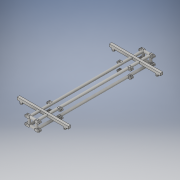
# Autodesk Inventor part: prototype body
Saved by Autodesk Inventor 2016 (Build 200138000, 138)
## iProperties
Created: 2017-06-26
Part Number: prototype body
Material: Generic
Document SubType Name: Modeling
Designer: andon
Density: 1 g/cm^3
Appearance: Default
Author: andon
Autodesk Inventor part; units mm, degrees
sketch "Sketch1" plane through (0, 0, 0) normal (0, 0, 1) x (1, 0, 0)
  line L0 (-76.2, -76.2) -> (76.2, -76.2)
  line L1 (76.2, -76.2) -> (76.2, 76.2)
  line L2 (76.2, 76.2) -> (-76.2, 76.2)
  line L3 (-76.2, 76.2) -> (-76.2, -76.2)
  line L4 (-76.2, -76.2) -> (76.2, 76.2) construction
  line L5 (76.2, -76.2) -> (-76.2, 76.2) construction
  circle A0 centre (-76.2, 76.2) radius 25.4
  circle A1 centre (76.2, 76.2) radius 25.4
  circle A2 centre (-76.2, -76.2) radius 25.4
  circle A3 centre (76.2, -76.2) radius 25.4
  point P0 (0, 0)
  dimension "d0" = 152.4
  dimension "d1" = 152.4
  dimension "d6" = 50.8
  constraints: 12 end point, 4 centre point, 4 coincident, 3 equal radius, 2 midpoint, 2 parallel, 1 horizontal, 1 perpendicular
  measures "d0" distance of L2.end L1.end
  measures "d1" distance of L1.end L0.end
  measures "d6" diameter of A1
sketch "Sketch1 outline for Extrusion1" plane through (0, 0, 0) normal (0, 0, 1) x (1, 0, 0)
  circle A0 centre (-76.2, 76.2) radius 25.4
  circle A1 centre (76.2, 76.2) radius 25.4
  circle A2 centre (-76.2, -76.2) radius 25.4
  circle A3 centre (76.2, -76.2) radius 25.4
extrude "Extrusion1" add sketch "Sketch1 outline for Extrusion1" along normal mid plane 2438.4
sketch "Sketch2" plane through (-76.2, 76.2, 1219.2) normal (0, 0, 1) x (1, 0, 0)
  circle A0 centre (0, 0) radius 25.4 projected
  circle A1 centre (0, -152.4) radius 25.4 projected
  circle A2 centre (152.4, 0) radius 25.4 projected
  circle A3 centre (152.4, -152.4) radius 25.4 projected
  line L0 (0, 0) -> (152.4, 0)
  line L1 (152.4, 0) -> (152.4, -152.4)
  line L2 (152.4, -152.4) -> (0, -152.4)
  line L3 (0, -152.4) -> (0, 0)
  point P0 (76.2, -76.2)
  constraints: 8 end point, 2 parallel, 1 horizontal, 1 perpendicular
ref_plane "Work Plane1" through (76.2, 76.2, 1219.2) normal (-1, 0, 0) x (0, -1, 0)
sketch "Sketch3" plane through (76.2, 76.2, 1219.2) normal (-1, 0, 0) x (0, -1, 0)
  circle A0 centre (0, -25.4) radius 25.4
  circle A1 centre (152.4, -25.4) radius 25.4
  line L0 (25.4, -1219.2) -> (-25.4, -1219.2) projected
  line L1 (25.4, -1219.2) -> (-25.4, -1219.2) projected
  line L2 (177.8, -1219.2) -> (127, -1219.2) projected
  circle A2 centre (152.4, -2413) radius 25.4
  line L3 (127, -2438.4) -> (127, 0) projected
  circle A3 centre (0, -2413) radius 25.4
  line L4 (-25.4, -2438.4) -> (-25.4, 0) projected
  point P0 (76.2, -1219.2)
  dimension "d10" = 50.8
  constraints: 4 centre point, 2 tangent, 1 equal radius
  measures "d10" diameter of A0
sketch "Sketch3 outline for Extrusion2" plane through (76.2, 76.2, 1219.2) normal (-1, 0, 0) x (0, -1, 0)
  circle A0 centre (0, -25.4) radius 25.4
  circle A1 centre (152.4, -25.4) radius 25.4
  circle A2 centre (152.4, -2413) radius 25.4
  circle A3 centre (0, -2413) radius 25.4
extrude "Extrusion2" add sketch "Sketch3 outline for Extrusion2" along normal blind 152.4
ref_plane "Work Plane2" through (-76.2, 76.2, 1219.2) normal (0, -1, 0) x (1, 0, 0)
sketch "Sketch4" plane through (-76.2, 76.2, 1219.2) normal (0, -1, 0) x (1, 0, 0)
  line L0 (0, -25.4) -> (25.4, -50.8) projected
  circle A0 centre (0, -25.4) radius 25.4
  line L1 (152.4, -25.4) -> (127, 0) projected
  circle A1 centre (152.4, -25.4) radius 25.4
  line L2 (0, -1803.4) -> (0, -1803.4) projected
  line L3 (152.4, -1803.4) -> (127, -1778) projected
  circle A2 centre (0, -2413) radius 25.4
  line L4 (-25.4, -2438.4) -> (25.4, -2438.4) projected
  line L5 (152.4, -2413) -> (127, -2387.6) projected
  circle A3 centre (152.4, -2413) radius 25.4
  point P0 (76.2, -1219.2)
  dimension "d14" = 50.8
  constraints: 4 centre point, 1 equal radius, 1 tangent, 1 other
  measures "d14" diameter of A0
sketch "Sketch4 outline for Extrusion3" plane through (-76.2, 76.2, 1219.2) normal (0, -1, 0) x (1, 0, 0)
  circle A0 centre (0, -25.4) radius 25.4
  circle A1 centre (152.4, -25.4) radius 25.4
  circle A2 centre (0, -2413) radius 25.4
  circle A3 centre (152.4, -2413) radius 25.4
extrude "Extrusion3" add sketch "Sketch4 outline for Extrusion3" along normal blind 152.4
ref_plane "Work Plane3" through (0, 76.2, 1219.2) normal (-1, 0, 0) x (0, -1, 0)
sketch "Sketch7" plane through (0, 76.2, 1219.2) normal (-1, 0, 0) x (0, -1, 0)
  line L0 (-25.4, -228.6) -> (25.4, -228.6)
  line L1 (25.4, -228.6) -> (25.4, -279.4)
  line L2 (25.4, -279.4) -> (-25.4, -279.4)
  line L3 (-25.4, -279.4) -> (-25.4, -228.6)
  line L4 (-25.4, -228.6) -> (25.4, -279.4) construction
  line L5 (25.4, -228.6) -> (-25.4, -279.4) construction
  point P0 (76.2, -1219.2)
  point P1 (0, -254)
  dimension "d23" = 50.8
  dimension "d24" = 50.8
  constraints: 12 end point, 2 midpoint, 2 parallel, 1 horizontal, 1 perpendicular
  measures "d23" distance of L1.end L2.end
  measures "d24" distance of L0.end L1.end
sketch "Sketch7 outline for Extrusion4" plane through (0, 76.2, 1219.2) normal (-1, 0, 0) x (0, -1, 0)
  line L0 (-25.4, -228.6) -> (25.4, -228.6)
  line L1 (25.4, -228.6) -> (25.4, -279.4)
  line L2 (25.4, -279.4) -> (-25.4, -279.4)
  line L3 (-25.4, -279.4) -> (-25.4, -228.6)
extrude "Extrusion4" add sketch "Sketch7 outline for Extrusion4" along normal mid plane 1066.8
sketch "Sketch9" plane through (76.2, 76.2, 1219.2) normal (-1, 0, 0) x (0, -1, 0)
  line L0 (0, -25.4) -> (25.4, -50.8) projected
  line L1 (-25.4, 0) -> (25.4, 0)
  line L2 (25.4, 0) -> (25.4, -50.8)
  line L3 (25.4, -50.8) -> (-25.4, -50.8)
  line L4 (-25.4, -50.8) -> (-25.4, 0)
  line L5 (-25.4, 0) -> (25.4, -50.8) construction
  line L6 (25.4, 0) -> (-25.4, -50.8) construction
  line L7 (127, 0) -> (177.8, 0)
  line L8 (177.8, 0) -> (177.8, -50.8)
  line L9 (177.8, -50.8) -> (127, -50.8)
  line L10 (127, -50.8) -> (127, 0)
  line L11 (152.4, -25.4) -> (127, 0) projected
  line L12 (127, 0) -> (177.8, -50.8) construction
  line L13 (177.8, 0) -> (127, -50.8) construction
  line L14 (-50.8, -25.4) -> (-50.8, -482.6)
  line L15 (-25.4, -457.2) -> (25.4, -457.2)
  line L16 (25.4, -457.2) -> (25.4, -508)
  line L17 (25.4, -508) -> (-25.4, -508)
  line L18 (-25.4, -508) -> (-25.4, -457.2)
  line L19 (-25.4, -457.2) -> (25.4, -508) construction
  line L20 (25.4, -457.2) -> (-25.4, -508) construction
  line L21 (127, -457.2) -> (177.8, -457.2)
  line L22 (177.8, -457.2) -> (177.8, -508)
  line L23 (177.8, -508) -> (127, -508)
  line L24 (127, -508) -> (127, -457.2)
  line L25 (127, -457.2) -> (177.8, -508) construction
  line L26 (177.8, -457.2) -> (127, -508) construction
  point P0 (76.2, -1219.2)
  point P1 (17.960512, -43.360512)
  point P2 (0, -482.6)
  point P3 (152.4, -482.6)
  dimension "d27" = 50.8
  dimension "d28" = 50.8
  dimension "d29" = 50.8
  dimension "d30" = 50.8
  dimension "d31" = 457.2
  dimension "d32" = 50.8
  dimension "d33" = 50.8
  dimension "d34" = 50.8
  dimension "d35" = 50.8
  constraints: 50 end point, 8 midpoint, 8 parallel, 4 horizontal, 4 perpendicular, 1 vertical
  measures "d27" distance of L0.end L3.end
  measures "d28" distance of L1.end L0.end
  measures "d29" distance of L8.end L9.end
  measures "d30" distance of L7.end L8.end
  measures "d31" distance of L14.start L14.end
  measures "d32" distance of L16.end L17.end
  measures "d33" distance of L15.end L16.end
  measures "d34" distance of L22.end L23.end
  measures "d35" distance of L21.end L22.end
sketch "Sketch9 outline for Extrusion5" plane through (76.2, 76.2, 1219.2) normal (-1, 0, 0) x (0, -1, 0)
  line L0 (-25.4, 0) -> (25.4, 0)
  line L1 (25.4, 0) -> (25.4, -50.8)
  line L2 (25.4, -50.8) -> (-25.4, -50.8)
  line L3 (-25.4, -50.8) -> (-25.4, 0)
  line L4 (127, 0) -> (177.8, 0)
  line L5 (177.8, 0) -> (177.8, -50.8)
  line L6 (177.8, -50.8) -> (127, -50.8)
  line L7 (127, -50.8) -> (127, 0)
  line L8 (-25.4, -457.2) -> (25.4, -457.2)
  line L9 (25.4, -457.2) -> (25.4, -508)
  line L10 (25.4, -508) -> (-25.4, -508)
  line L11 (-25.4, -508) -> (-25.4, -457.2)
  line L12 (127, -457.2) -> (177.8, -457.2)
  line L13 (177.8, -457.2) -> (177.8, -508)
  line L14 (177.8, -508) -> (127, -508)
  line L15 (127, -508) -> (127, -457.2)
extrude "Extrusion5" add sketch "Sketch9 outline for Extrusion5" against normal blind 76.2
sketch "Sketch10" plane through (152.4, 76.2, 1219.2) normal (1, 0, 0) x (0, 0, -1)
  line L0 (50.8, 25.4) -> (0, 25.4) projected
  line L1 (0, -25.4) -> (50.8, -25.4) projected
  line L2 (12.7, 25.4) -> (38.1, 25.4)
  line L3 (38.1, 25.4) -> (38.1, -25.4)
  line L4 (38.1, -25.4) -> (12.7, -25.4)
  line L5 (12.7, -25.4) -> (12.7, 25.4)
  line L6 (50.8, -127) -> (0, -127) projected
  line L7 (2438.4, -177.8) -> (0, -177.8) projected
  line L8 (12.7, -127) -> (38.1, -127)
  line L9 (38.1, -127) -> (38.1, -177.8)
  line L10 (38.1, -177.8) -> (12.7, -177.8)
  line L11 (12.7, -177.8) -> (12.7, -127)
  line L12 (2387.6, -127) -> (50.8, -127) projected
  line L13 (469.9, -127) -> (495.3, -127)
  line L14 (495.3, -127) -> (495.3, -177.8)
  line L15 (495.3, -177.8) -> (469.9, -177.8)
  line L16 (469.9, -177.8) -> (469.9, -127)
  line L17 (2387.6, -25.4) -> (279.4, -25.4) projected
  line L18 (469.9, 25.4) -> (495.3, 25.4)
  line L19 (495.3, 25.4) -> (495.3, -25.4)
  line L20 (495.3, -25.4) -> (469.9, -25.4)
  line L21 (469.9, -25.4) -> (469.9, 25.4)
  point P0 (1219.2, -76.2)
  constraints: 32 end point, 12 point on line, 8 parallel, 4 horizontal, 4 perpendicular
sketch "Sketch10 outline for Extrusion6" plane through (152.4, 76.2, 1219.2) normal (1, 0, 0) x (0, 0, -1)
  line L0 (12.7, 25.4) -> (38.1, 25.4)
  line L1 (38.1, 25.4) -> (38.1, -25.4)
  line L2 (38.1, -25.4) -> (12.7, -25.4)
  line L3 (12.7, -25.4) -> (12.7, 25.4)
  line L4 (469.9, 25.4) -> (495.3, 25.4)
  line L5 (495.3, 25.4) -> (495.3, -25.4)
  line L6 (495.3, -25.4) -> (469.9, -25.4)
  line L7 (469.9, -25.4) -> (469.9, 25.4)
  line L8 (469.9, -177.8) -> (495.3, -177.8)
  line L9 (469.9, -127) -> (469.9, -177.8)
  line L10 (495.3, -127) -> (469.9, -127)
  line L11 (495.3, -177.8) -> (495.3, -127)
  line L12 (38.1, -127) -> (12.7, -127)
  line L13 (38.1, -177.8) -> (38.1, -127)
  line L14 (12.7, -177.8) -> (38.1, -177.8)
  line L15 (12.7, -127) -> (12.7, -177.8)
extrude "Extrusion6" cut sketch "Sketch10 outline for Extrusion6" against normal blind 50.8
fillet "Fillet1" radius 25.4 16 edges at (152.4, 101.6, 1212.85) (152.4, 50.8, 1212.85) (152.4, 50.8, 1174.75) (152.4, 101.6, 1174.75) (152.4, -50.8, 1174.75) (152.4, -101.6, 1174.75) (152.4, -101.6, 1212.85) (152.4, -50.8, 1212.85) (152.4, 101.6, 755.65) (152.4, 101.6, 717.55) (152.4, 50.8, 717.55) (152.4, 50.8, 755.65) (152.4, -50.8, 755.65) (152.4, -50.8, 717.55) (152.4, -101.6, 717.55) (152.4, -101.6, 755.65)
sketch "Sketch11" plane through (0, 0, 1219.2) normal (0, 0, 1) x (1, 0, 0)
  arc A0 (127, 50.8) -> (127, 101.6) centre (127, 76.2) ccw projected
  circle A1 centre (127, 76.2) radius 9.525
  circle A2 centre (127, -76.2) radius 9.525
  point P0 (0, 0)
  constraints: 2 centre point, 1 coincident
sketch "Sketch11 outline for Extrusion7" plane through (0, 0, 1219.2) normal (0, 0, 1) x (1, 0, 0)
  circle A0 centre (127, 76.2) radius 9.525
  circle A1 centre (127, -76.2) radius 9.525
extrude "Extrusion7" cut sketch "Sketch11 outline for Extrusion7" against normal blind 76.2
sketch "Sketch12" plane through (76.2, 76.2, 762) normal (0, 0, 1) x (1, 0, 0)
  circle A0 centre (50.8, 0) radius 9.525 projected
  circle A1 centre (50.8, -152.4) radius 9.525 projected
  point P0 (-76.2, -76.2)
sketch "Sketch12 outline for Extrusion8" plane through (76.2, 76.2, 762) normal (0, 0, 1) x (1, 0, 0)
  circle A0 centre (50.8, 0) radius 9.525
  circle A1 centre (50.8, -152.4) radius 9.525
extrude "Extrusion8" cut sketch "Sketch12 outline for Extrusion8" against normal blind 76.2
mirror "Mirror1" about plane through (0, 76.2, 1219.2) normal (-1, 0, 0) of "Extrusion5", "Fillet1", "Extrusion7", "Extrusion8", "Extrusion6"
ref_plane "Work Plane4" through (0, 0, 0) normal (0, 0, 1) x (1, 0, 0)
mirror "Mirror2" about plane through (0, 0, 0) normal (0, 0, 1) of "Extrusion4", "Extrusion5", "Fillet1", "Extrusion7", "Extrusion8", "Extrusion6", "Mirror1"
sketch "Sketch13" plane through (-533.4, 50.8, 990.6) normal (0, -1, 0) x (1, 0, 0)
  line L0 (1016, 0) -> (1016, -50.8)
  line L1 (1016, 0) -> (965.2, 0)
  line L2 (965.2, 0) -> (965.2, -50.8)
  line L3 (965.2, -50.8) -> (1016, -50.8)
  line L4 (1016, -50.8) -> (1016, 0)
  line L5 (0, 0) -> (457.2, 0) projected
  line L6 (101.6, 0) -> (50.8, 0)
  line L7 (50.8, 0) -> (50.8, -50.8)
  line L8 (50.8, -50.8) -> (101.6, -50.8)
  line L9 (101.6, -50.8) -> (101.6, 0)
  line L10 (0, -1930.4) -> (457.2, -1930.4) projected
  line L11 (457.2, -1981.2) -> (0, -1981.2) projected
  line L12 (50.8, -1930.4) -> (101.6, -1930.4)
  line L13 (101.6, -1930.4) -> (101.6, -1981.2)
  line L14 (101.6, -1981.2) -> (50.8, -1981.2)
  line L15 (50.8, -1981.2) -> (50.8, -1930.4)
  line L16 (609.6, -1930.4) -> (1066.8, -1930.4) projected
  line L17 (609.6, -1981.2) -> (1066.8, -1981.2) projected
  line L18 (965.2, -1930.4) -> (1016, -1930.4)
  line L19 (1016, -1930.4) -> (1016, -1981.2)
  line L20 (1016, -1981.2) -> (965.2, -1981.2)
  line L21 (965.2, -1981.2) -> (965.2, -1930.4)
  point P0 (533.4, -990.6)
  point P1 (1066.8, 0)
  dimension "d49" = 50.8
  dimension "d50" = 50.8
  constraints: 34 end point, 8 parallel, 7 point on line, 4 horizontal, 4 perpendicular
  measures "d49" distance of L8.end L7.end
  measures "d50" distance of L7.end L6.end
sketch "Sketch13 outline for Extrusion9" plane through (-533.4, 50.8, 990.6) normal (0, -1, 0) x (1, 0, 0)
  line L0 (1016, -50.8) -> (1016, 0)
  line L1 (965.2, -50.8) -> (1016, -50.8)
  line L2 (965.2, 0) -> (965.2, -50.8)
  line L3 (1016, 0) -> (965.2, 0)
  line L4 (101.6, -50.8) -> (101.6, 0)
  line L5 (50.8, -50.8) -> (101.6, -50.8)
  line L6 (50.8, 0) -> (50.8, -50.8)
  line L7 (101.6, 0) -> (50.8, 0)
  line L8 (50.8, -1930.4) -> (101.6, -1930.4)
  line L9 (101.6, -1930.4) -> (101.6, -1981.2)
  line L10 (101.6, -1981.2) -> (50.8, -1981.2)
  line L11 (50.8, -1981.2) -> (50.8, -1930.4)
  line L12 (965.2, -1930.4) -> (1016, -1930.4)
  line L13 (1016, -1930.4) -> (1016, -1981.2)
  line L14 (1016, -1981.2) -> (965.2, -1981.2)
  line L15 (965.2, -1981.2) -> (965.2, -1930.4)
extrude "Extrusion9" add sketch "Sketch13 outline for Extrusion9" along normal blind 50.8
sketch "Sketch14" plane through (-533.4, 0, 990.6) normal (0, -1, 0) x (1, 0, 0)
  line L0 (50.8, -50.8) -> (50.8, 0) projected
  line L1 (101.6, 0) -> (101.6, -50.8) projected
  line L2 (50.8, -12.7) -> (101.6, -12.7)
  line L3 (101.6, -12.7) -> (101.6, -38.1)
  line L4 (101.6, -38.1) -> (50.8, -38.1)
  line L5 (50.8, -38.1) -> (50.8, -12.7)
  line L6 (1016, -50.8) -> (1016, 0) projected
  line L7 (965.2, -12.7) -> (1016, -12.7)
  line L8 (1016, -12.7) -> (1016, -38.1)
  line L9 (1016, -38.1) -> (965.2, -38.1)
  line L10 (965.2, -38.1) -> (965.2, -12.7)
  line L11 (965.2, -1930.4) -> (965.2, -1981.2) projected
  line L12 (1016, -1930.4) -> (1016, -1981.2) projected
  line L13 (965.2, -1943.1) -> (1016, -1943.1)
  line L14 (1016, -1943.1) -> (1016, -1968.5)
  line L15 (1016, -1968.5) -> (965.2, -1968.5)
  line L16 (965.2, -1968.5) -> (965.2, -1943.1)
  line L17 (50.8, -1930.4) -> (50.8, -1981.2) projected
  line L18 (101.6, -1943.1) -> (50.8, -1943.1)
  line L19 (50.8, -1943.1) -> (50.8, -1968.5)
  line L20 (50.8, -1968.5) -> (101.6, -1968.5)
  line L21 (101.6, -1968.5) -> (101.6, -1943.1)
  point P0 (533.4, -990.6)
  constraints: 32 end point, 11 point on line, 8 parallel, 4 horizontal, 4 perpendicular
sketch "Sketch14 outline for Extrusion10" plane through (-533.4, 0, 990.6) normal (0, -1, 0) x (1, 0, 0)
  line L0 (50.8, -12.7) -> (101.6, -12.7)
  line L1 (101.6, -12.7) -> (101.6, -38.1)
  line L2 (101.6, -38.1) -> (50.8, -38.1)
  line L3 (50.8, -38.1) -> (50.8, -12.7)
  line L4 (965.2, -12.7) -> (1016, -12.7)
  line L5 (1016, -12.7) -> (1016, -38.1)
  line L6 (1016, -38.1) -> (965.2, -38.1)
  line L7 (965.2, -38.1) -> (965.2, -12.7)
  line L8 (965.2, -1943.1) -> (1016, -1943.1)
  line L9 (1016, -1943.1) -> (1016, -1968.5)
  line L10 (1016, -1968.5) -> (965.2, -1968.5)
  line L11 (965.2, -1968.5) -> (965.2, -1943.1)
  line L12 (101.6, -1968.5) -> (101.6, -1943.1)
  line L13 (50.8, -1968.5) -> (101.6, -1968.5)
  line L14 (50.8, -1943.1) -> (50.8, -1968.5)
  line L15 (101.6, -1943.1) -> (50.8, -1943.1)
extrude "Extrusion10" cut sketch "Sketch14 outline for Extrusion10" against normal blind 38.1
fillet "Fillet2" radius 25.4 16 edges at (482.6, 0, 984.25) (482.6, 0, 946.15) (431.8, 0, 984.25) (431.8, 0, 946.15) (-482.6, 0, 984.25) (-482.6, 0, 946.15) (-431.8, 0, 984.25) (-431.8, 0, 946.15) (-431.8, 0, -946.15) (-431.8, 0, -984.25) (-482.6, 0, -984.25) (-482.6, 0, -946.15) (431.8, 0, -946.15) (431.8, 0, -984.25) (482.6, 0, -946.15) (482.6, 0, -984.25)
sketch "Sketch15" plane through (76.2, 101.6, 990.6) normal (0, 0, 1) x (1, 0, 0)
  arc A0 (355.6, -76.2) -> (406.4, -76.2) centre (381, -76.2) ccw projected
  circle A1 centre (381, -76.2) radius 9.525
  arc A2 (-558.8, -76.2) -> (-508, -76.2) centre (-533.4, -76.2) ccw projected
  circle A3 centre (-533.4, -76.2) radius 9.525
  point P0 (-76.2, -101.6)
  constraints: 2 centre point, 2 coincident
sketch "Sketch15 outline for Extrusion11" plane through (76.2, 101.6, 990.6) normal (0, 0, 1) x (1, 0, 0)
  circle A0 centre (381, -76.2) radius 9.525
  circle A1 centre (-533.4, -76.2) radius 9.525
extrude "Extrusion11" cut sketch "Sketch15 outline for Extrusion11" against normal blind 2540
body "Solid1"
